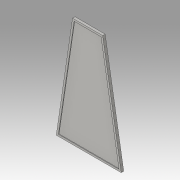
# Autodesk Inventor part: GearProtector
Saved by Autodesk Inventor 2016 (Build 200138000, 138)
## iProperties
Created: 2017-02-15
Part Number: GearProtector
Material: Generic
Document SubType Name: Modeling
Designer: Delta
Density: 1 g/cm^3
Appearance: Default
Author: Delta
Autodesk Inventor part; units mm, degrees
ref_plane "YZ Plane" through (0, 0, 0) normal (1, 0, 0) x (0, 1, 0)
ref_plane "XZ Plane" through (0, 0, 0) normal (0, 1, 0) x (-1, 0, 0)
ref_plane "XY Plane" through (0, 0, 0) normal (0, 0, 1) x (1, 0, 0)
sketch "Sketch1" plane through (0, 0, 0) normal (0, 0, 1) x (1, 0, 0)
  line L0 (0, 0) -> (88.9, 0)
  line L1 (22.225, 149.86) -> (63.5, 149.86)
  line L2 (63.5, 149.86) -> (88.9, 0)
  line L3 (0, 0) -> (22.225, 149.86)
  dimension "d0" = 88.9
  dimension "d1" = 41.275
  constraints: 8 end point, 2 horizontal
  measures "d0" distance of L0.start L0.end
  measures "d1" distance of L1.start L1.end
extrude "Extrusion1" add sketch "Sketch1" along normal blind 3.429
shell "Shell1" thickness 2.54 removed faces 1 at (50.8, 49.9533, 3.429)
shell "Shell2" thickness 1.27 removed faces 1 at (50.064, 50.8, 2.54)
shell "Shell3" thickness 0.508 removed faces 1 at (50.432, 50.3767, 1.27)
body "Solid1"
